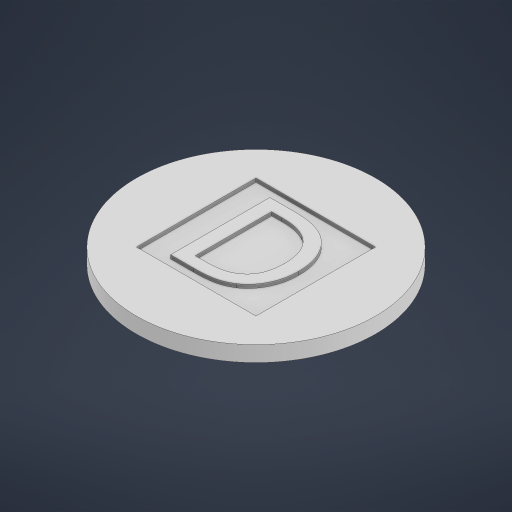
# Autodesk Inventor part: TopMarkerPreset
Saved by Autodesk Inventor 2023.2 (Build 272271030, 271C)
## iProperties
Created: 2023-05-05
Part Number: TopMarkerPreset
Material: Generic
Document SubType Name: Modeling
Designer: Elias Braun
Density: 1 g/cm^3
Appearance: Default
Author: Elias Braun
Autodesk Inventor part; units mm, degrees
ref_plane "YZ Plane" through (0, 0, 0) normal (1, 0, 0) x (0, 1, 0)
ref_plane "XZ Plane" through (0, 0, 0) normal (0, 1, 0) x (-1, 0, 0)
ref_plane "XY Plane" through (0, 0, 0) normal (0, 0, 1) x (1, 0, 0)
sketch "Sketch1" plane through (0, 0, 0) normal (0, 1, 0) x (-1, 0, 0)
  circle A0 centre (0, 0) radius 20
  dimension "d0" = 40
  constraints: 1 centre point, 1 coincident
  measures "d0" diameter of A0
extrude "Extrusion1" add sketch "Sketch1" along normal blind 2.6
sketch "Sketch2" plane through (0, 2.6, 0) normal (0, 1, 0) x (1, 0, 0)
  line L0 (-10, -10) -> (-10, 10)
  line L1 (-10, 10) -> (10, 10)
  line L2 (10, 10) -> (10, -10)
  line L3 (10, -10) -> (-10, -10)
  line L4 (-10, -10) -> (10, 10) construction
  line L5 (-10, 10) -> (10, -10) construction
  point P0 (0, 0)
  dimension "d3" = 20
  dimension "d4" = 20
  constraints: 12 end point, 2 midpoint, 2 parallel, 1 perpendicular, 1 vertical
  measures "d3" distance of L0.start L0.end
  measures "d4" distance of L0.end L1.end
extrude "Extrusion2" cut sketch "Sketch2" against normal blind 0.6
sketch "Sketch3" plane through (0, 2, 0) normal (0, 1, 0) x (1, 0, 0)
  line L0 (-7.7054, 8.3364) -> (7.7781, 8.3364) construction
  line L1 (7.7781, 8.3364) -> (7.7781, -8.2636) construction
  line L2 (7.7781, -8.2636) -> (-7.7054, -8.2636) construction
  line L3 (-7.7054, -8.2636) -> (-7.7054, 8.3364) construction
  spline S0 degree 2 poles (7.0651, 0.0229) (7.0651, -2.2505) (5.2222, -5.9095) (3.6752, -6.9319) knots 0 0 0 1 2 2 2
  spline S1 degree 2 poles (3.6752, -6.9319) (2.4107, -7.7256) (-0.1856, -8.2636) (-2.2034, -8.2636) knots 0 0 0 1 2 2 2
  line L4 (-2.2034, -8.2636) -> (-6.0239, -8.2636)
  line L5 (-6.0239, -8.2636) -> (-6.0239, 8.3364)
  line L6 (-6.0239, 8.3364) -> (-2.2438, 8.3364)
  spline S2 degree 2 poles (-2.2438, 8.3364) (0.0969, 8.3364) (2.7604, 7.6368) (3.7021, 7.018) knots 0 0 0 1 2 2 2
  spline S3 degree 2 poles (3.7021, 7.018) (5.3029, 5.9553) (7.0651, 2.4443) (7.0651, 0.0229) knots 0 0 0 1 2 2 2
  spline S4 degree 2 poles (4.7648, 0.0498) (4.7648, 1.96) (3.5003, 4.6639) (2.2492, 5.4307) knots 0 0 0 1 2 2 2
  spline S5 degree 2 poles (2.2492, 5.4307) (1.3614, 5.9553) (-0.643, 6.4261) (-2.1362, 6.4261) knots 0 0 0 1 2 2 2
  line L7 (-2.1362, 6.4261) -> (-3.8177, 6.4261)
  line L8 (-3.8177, 6.4261) -> (-3.8177, -6.3534)
  line L9 (-3.8177, -6.3534) -> (-2.1362, -6.3534)
  spline S6 degree 2 poles (-2.1362, -6.3534) (-0.6699, -6.3534) (1.5497, -5.8826) (2.451, -5.2504) knots 0 0 0 1 2 2 2
  spline S7 degree 2 poles (2.451, -5.2504) (3.6079, -4.4701) (4.7648, -1.8873) (4.7648, 0.0498) knots 0 0 0 1 2 2 2
  point P0 (0, 0)
  constraints: 2 other
extrude "Extrusion3" add sketch "Sketch3" along normal blind 0.6
body "Solid1"
